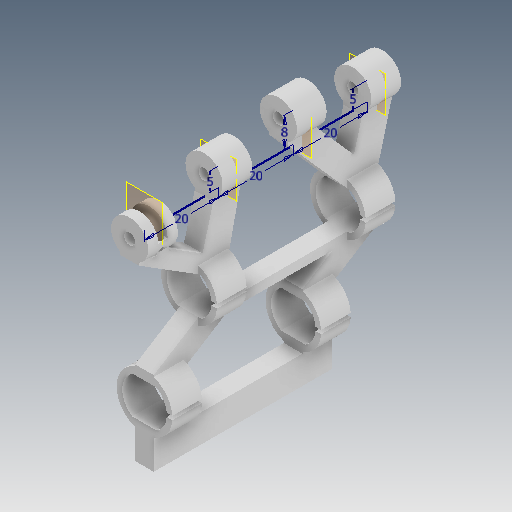
# Autodesk Inventor part: base_hand
Saved by Autodesk Inventor 2020.2 (Build 242310000, 310)
## iProperties
Created: 2020-04-08
Part Number: base_hand
Material: Generic
Document SubType Name: Modeling
Designer: Bardo91
Density: 1 g/cm^3
Appearance: Default
Author: Bardo91
Autodesk Inventor part; units mm, degrees
ref_plane "YZ Plane" through (0, 0, 0) normal (1, 0, 0) x (0, 1, 0)
ref_plane "XZ Plane" through (0, 0, 0) normal (0, 1, 0) x (-1, 0, 0)
sketch "Sketch1" plane through (0, 0, 0) normal (1, 0, 0) x (0, 1, 0)
  line L0 (0, 0) -> (0, -20)
  line L1 (0, -20) -> (0, -40)
  line L2 (0, -40) -> (0, -60)
  line L3 (0, -20) -> (5, -20)
  line L4 (0, -40) -> (8, -40)
  line L5 (0, -60) -> (5, -60)
  dimension "d0" = 20
  dimension "d1" = 20
  dimension "d2" = 20
  dimension "d4" = 5
  dimension "d5" = 8
  dimension "d6" = 5
  constraints: 12 end point, 2 horizontal, 2 point on line, 1 perpendicular, 1 vertical
  measures "d0" distance of L0.start L0.end
  measures "d1" distance of L0.end L1.end
  measures "d2" distance of L1.end L2.end
  measures "d4" distance of L0.end L3.end
  measures "d5" distance of L1.end L4.end
  measures "d6" distance of L2.end L5.end
ref_plane "Work Plane1" through (0, 5, -20) normal (0, 0, 1) x (1, 0, 0)
ref_plane "Work Plane3" through (0, 5, -60) normal (0, 0, 1) x (1, 0, 0)
ref_plane "Work Plane2" through (0, 8, -40) normal (0, 0, 1) x (1, 0, 0)
ref_plane "Work Plane4" through (0, 0, 0) normal (0, 0, 1) x (1, 0, 0)
sketch "Sketch2" plane through (0, 0, 0) normal (0, 0, 1) x (1, 0, 0)
  circle A0 centre (0, 0) radius 1.5
  circle A1 centre (0, 0) radius 5
  dimension "d7" = 3
  dimension "d8" = 10
  constraints: 2 centre point, 2 coincident
  measures "d7" diameter of A0
  measures "d8" diameter of A1
sketch "Sketch3" plane through (0, 5, -20) normal (0, 0, 1) x (1, 0, 0)
  circle A0 centre (0, 0) radius 1.5
  circle A1 centre (0, 0) radius 5
  point P0 (0, -5)
  dimension "d9" = 3
  dimension "d10" = 10
  constraints: 2 centre point, 1 coincident
  measures "d9" diameter of A0
  measures "d10" diameter of A1
sketch "Sketch4" plane through (0, 8, -40) normal (0, 0, 1) x (1, 0, 0)
  circle A0 centre (0, 0) radius 1.5
  circle A1 centre (0, 0) radius 5
  point P0 (0, -8)
  dimension "d11" = 3
  dimension "d12" = 10
  constraints: 2 centre point, 1 coincident
  measures "d11" diameter of A0
  measures "d12" diameter of A1
sketch "Sketch5" plane through (0, 5, -60) normal (0, 0, 1) x (1, 0, 0)
  circle A0 centre (0, 0) radius 1.5
  circle A1 centre (0, 0) radius 5
  point P0 (0, -5)
  dimension "d13" = 3
  dimension "d14" = 10
  constraints: 2 centre point, 1 coincident
  measures "d13" diameter of A0
  measures "d14" diameter of A1
extrude "pinky_joint" add sketch "Sketch2" along normal mid plane 8
extrude "ring_joint" add sketch "Sketch3" along normal mid plane 8
extrude "middle_joint" add sketch "Sketch4" along normal mid plane 8
extrude "index_joint" add sketch "Sketch5" along normal mid plane 8
sketch "Sketch6" plane through (0, 0, 0) normal (0, 0, 1) x (1, 0, 0)
  circle A0 centre (0, 0) radius 1.5 projected
  line L0 (0, 0) -> (0, -20)
  line L1 (0, -20) -> (0, -40)
  circle A1 centre (0, -40) radius 6
  circle A2 centre (0, -40) radius 7.5
  line L2 (0, -40) -> (0, -35)
  line L3 (0, -35) -> (3.3166, -35)
  line L4 (0, -35) -> (-3.3166, -35)
  line L5 (0, -40) -> (0, -45)
  line L6 (0, -45) -> (3.3166, -45)
  line L7 (0, -45) -> (-3.3166, -45)
  line L8 (0, -40) -> (0, -40.5)
  line L9 (0, -40) -> (0, -39.5)
  line L10 (0, -39.5) -> (7.4833, -39.5)
  line L11 (0, -40.5) -> (7.4833, -40.5)
  point P0 (5.9791, -39.5)
  point P1 (5.9791, -40.5)
  dimension "d23" = 20
  dimension "d24" = 20
  dimension "d25" = 12
  dimension "d26" = 15
  dimension "d27" = 5
  dimension "d28" = 5
  dimension "d29" = 0.5
  dimension "d30" = 0.5
  constraints: 24 end point, 7 point on line, 6 point on circle, 3 perpendicular, 2 centre point, 2 coincident, 1 parallel, 1 vertical
  measures "d23" distance of L0.start L0.end
  measures "d24" distance of L0.end L1.end
  measures "d25" diameter of A1
  measures "d26" diameter of A2
  measures "d27" distance of L2.start L2.end
  measures "d28" distance of L2.start L5.end
  measures "d29" distance of L2.start L8.end
  measures "d30" distance of L2.start L9.end
extrude "ring_motor" add sketch "Sketch6" against normal blind 8 contours L4 A1 L1 | L1 A1 L3 | A1 L11 A2 L1 | L1 A2 L10 A1 | L7 L6 A1
sketch "Sketch7" plane through (0, 5, -20) normal (0, 0, 1) x (1, 0, 0)
  circle A0 centre (0, -5) radius 5 projected
  line L0 (0, -5) -> (0, -25)
  circle A1 centre (0, -25) radius 6
  circle A2 centre (0, -25) radius 7.5
  line L1 (0, -25) -> (0, -24.5)
  line L2 (0, -25) -> (0, -25.5)
  line L3 (0, -25.5) -> (7.4833, -25.5)
  line L4 (0, -24.5) -> (7.4833, -24.5)
  line L5 (0, -25) -> (0, -20)
  line L6 (0, -20) -> (3.3166, -20)
  line L7 (0, -20) -> (-3.3166, -20)
  line L8 (0, -25) -> (0, -30)
  line L9 (0, -30) -> (3.3166, -30)
  line L10 (0, -30) -> (-3.3166, -30)
  point P0 (5.9791, -24.5)
  point P1 (5.9791, -25.5)
  dimension "d33" = 20
  dimension "d34" = 12
  dimension "d35" = 15
  dimension "d36" = 0.5
  dimension "d37" = 0.5
  dimension "d50" = 5
  dimension "d51" = 5
  constraints: 22 end point, 6 point on circle, 5 point on line, 3 perpendicular, 2 centre point, 2 coincident, 2 vertical
  measures "d33" distance of L0.start L0.end
  measures "d34" diameter of A1
  measures "d35" diameter of A2
  measures "d36" distance of L1.start L1.end
  measures "d37" distance of L1.start L2.end
  measures "d50" distance of L1.start L5.end
  measures "d51" distance of L1.start L8.end
extrude "pinky_motor" add sketch "Sketch7" along normal blind 8 contours L7 A1 L0 | L0 A1 L6 | A1 L3 A2 L0 | L0 A2 L4 A1 | L10 L9 A1
sketch "Sketch8" plane through (0, 8, -40) normal (0, 0, 1) x (1, 0, 0)
  circle A0 centre (0, -8) radius 1.5 projected
  arc A1 (5.9791, -27.5) -> (5.9791, -28.5) centre (0, -28) ccw projected
  line L0 (0, -8) -> (0, -28)
  line L1 (0, -28) -> (0, -48)
  circle A2 centre (0, -48) radius 6
  circle A3 centre (0, -48) radius 7.5
  line L2 (0, -48) -> (0, -48.5)
  line L3 (5.9791, -48.5) -> (7.4833, -48.5) projected
  line L4 (0, -48.5) -> (7.4833, -48.5)
  line L5 (0, -48) -> (0, -47.5)
  arc A4 (7.4833, -47.5) -> (7.4833, -48.5) centre (0, -48) ccw projected
  line L6 (0, -47.5) -> (7.4833, -47.5)
  line L7 (0, -48) -> (0, -53)
  line L8 (0, -53) -> (3.3166, -53)
  arc A5 (5.9791, -47.5) -> (5.9791, -48.5) centre (0, -48) ccw projected
  line L9 (0, -53) -> (-3.3166, -53)
  line L10 (0, -48) -> (0, -43)
  line L11 (0, -43) -> (-3.3166, -43)
  line L12 (0, -43) -> (3.3166, -43)
  point P0 (3.3166, -53)
  point P1 (-3.3166, -53)
  point P2 (-3.3166, -43)
  point P3 (3.3166, -43)
  point P4 (0.7483, -48)
  point P5 (0, -48)
  point P6 (0, -48)
  point P7 (-5.4544, -45.5)
  point P8 (6.4575, -44.1854)
  point P9 (6, -43.5)
  point P10 (5.9867, -43.5)
  point P11 (5.4544, -45.5)
  point P12 (-5.9812, -43.475)
  point P13 (5.9955, -43.4941)
  dimension "d40" = 20
  dimension "d41" = 20
  dimension "d42" = 12
  dimension "d43" = 15
  dimension "d44" = 0.5
  dimension "d45" = 0.5
  dimension "d46" = 5
  dimension "d47" = 5
  constraints: 24 end point, 5 point on line, 4 point on circle, 2 centre point, 2 coincident, 2 perpendicular, 2 vertical, 1 horizontal
  measures "d40" distance of L0.start L0.end
  measures "d41" distance of L0.end L1.end
  measures "d42" diameter of A2
  measures "d43" diameter of A3
  measures "d44" distance of L2.start L2.end
  measures "d45" distance of L2.start L5.end
  measures "d46" distance of L7.start L7.end
  measures "d47" distance of L10.start L10.end
extrude "index_motor" add sketch "Sketch8" against normal blind 8 contours L11 A2 L1 | L1 A2 L12 | A2 L3 A3 L1 | L1 A3 L6 A2 | L9 L8 A2
sketch "Sketch9" plane through (0, 5, -60) normal (0, 0, 1) x (1, 0, 0)
  line L0 (0, -5) -> (0, -25)
  circle A0 centre (0, -25) radius 6
  circle A1 centre (0, -25) radius 7.5
  line L1 (0, -25) -> (0, -30)
  line L2 (3.3166, -30) -> (-3.3166, -30) projected
  line L3 (0, -30) -> (3.3166, -30)
  line L4 (3.3166, -30) -> (0, -30)
  line L5 (-3.3166, -30) -> (0, -30)
  line L6 (0, -25) -> (0, -20)
  line L7 (-3.3166, -20) -> (3.3166, -20) projected
  line L8 (0, -20) -> (3.3166, -20)
  line L9 (0, -20) -> (-3.3166, -20)
  line L10 (0, -25) -> (0, -25.5)
  line L11 (7.4833, -25.5) -> (5.9791, -25.5) projected
  line L12 (0, -25.5) -> (7.4833, -25.5)
  line L13 (0, -25) -> (0, -24.5)
  arc A2 (7.4833, -24.5) -> (7.4833, -25.5) centre (0, -25) ccw projected
  line L14 (0, -24.5) -> (7.4833, -24.5)
  point P0 (5.9791, -24.5)
  dimension "d52" = 20
  dimension "d53" = 12
  dimension "d54" = 15
  dimension "d55" = 5
  dimension "d56" = 5
  dimension "d57" = 0.5
  dimension "d58" = 0.5
  constraints: 24 end point, 3 point on line, 2 centre point, 2 coincident, 2 collinear, 2 vertical, 1 midpoint, 1 perpendicular, 1 point on circle
  measures "d52" distance of L0.start L0.end
  measures "d53" diameter of A0
  measures "d54" diameter of A1
  measures "d55" distance of L1.start L1.end
  measures "d56" distance of L1.start L6.end
  measures "d57" distance of L1.start L10.end
  measures "d58" distance of L1.start L13.end
extrude "middle_motor" add sketch "Sketch9" along normal blind 8 contours L7 A0 L0 | L0 A0 L7 | A0 L11 A1 L0 | L0 A1 L14 A0 | L2 A0
sketch "Sketch16" plane through (0, 0, 0) normal (1, 0, 0) x (0, 1, 0)
  line L0 (-15, -20) -> (-15, -12) projected
  line L1 (-19.5, -12) -> (-15, -12) projected
  line L2 (-19.5, -20) -> (-15, -20) projected
  line L3 (-15, -20) -> (3.5, -24)
  line L4 (0, -24) -> (10, -24) projected
  line L5 (-15, -60) -> (-15, -52) projected
  line L6 (6.5, -36) -> (9.5, -36) projected
  line L7 (0, -64) -> (10, -64) projected
  line L8 (-5, -4) -> (5, -4) projected
  line L9 (-15, -20) -> (-5, -4)
  line L10 (10, -16) -> (0, -16) projected
  line L11 (-15, -12) -> (0, -16)
  line L12 (10, -56) -> (0, -56) projected
  line L13 (-15, -52) -> (0, -56)
  line L14 (3, -44) -> (13, -44) projected
  line L15 (3, -44) -> (-15, -60)
  line L16 (-5, -4) -> (-1.5, -4)
  line L17 (-1.5, 4) -> (-1.5, -4)
  line L18 (5, 4) -> (-5, 4) projected
  line L19 (0, -16) -> (3.5, -16)
  line L20 (6.5, -24) -> (3.5, -24) projected
  line L21 (3.5, -16) -> (3.5, -24)
  line L22 (3, -44) -> (6.5, -44)
  line L23 (-15, -12) -> (-5, 4)
  line L24 (-1.5, 4) -> (-5, 4)
  line L25 (9.5, -44) -> (6.5, -44) projected
  line L26 (3, -44) -> (6.5, -44)
  line L27 (6.5, -44) -> (6.5, -36)
  line L28 (13, -36) -> (3, -36) projected
  line L29 (3, -36) -> (6.5, -36)
  line L30 (3, -36) -> (-15, -52)
  line L31 (0, -56) -> (3.5, -56)
  line L32 (3.5, -64) -> (3.5, -56)
  line L33 (3.5, -56) -> (3.5, -64) projected
  line L34 (0, -64) -> (-15, -60)
  line L35 (-45, 0) -> (-45, -8) projected
  line L36 (-45, 0) -> (-55, 0)
  line L37 (-55, 0) -> (-55, -48)
  line L38 (-47.5, -48) -> (-32.5, -48) projected
  line L39 (-55, -48) -> (-45, -48)
  line L40 (-32.5, -40) -> (-47.5, -40) projected
  line L41 (-47.5, -8) -> (-32.5, -8) projected
  line L42 (-47.5, -40) -> (-47.5, -8)
  line L43 (-47.5, -8) -> (-45, -8)
  line L44 (-45, 0) -> (-40.5, 0) projected
  line L45 (-45, 0) -> (-45, -8)
  line L46 (-45, -40) -> (-45, -48) projected
  line L47 (-47.5, -40) -> (-45, -40)
  line L48 (-45, -40) -> (-45, -48)
  line L49 (-32.5, 0) -> (-47.5, 0) projected
  line L50 (-25, -20) -> (-25, -12) projected
  line L51 (-32.5, 0) -> (-25, -12)
  line L52 (-12.5, -20) -> (-27.5, -20) projected
  line L53 (-27.5, -20) -> (-35, -8)
  line L54 (-35, 0) -> (-35, -8) projected
  line L55 (-35, -8) -> (-35, 0)
  line L56 (-35, 0) -> (-32.5, 0)
  line L57 (-25, -12) -> (-20.5, -12) projected
  line L58 (-25, -12) -> (-25, -20)
  line L59 (-27.5, -20) -> (-25, -20)
  line L60 (-25, -60) -> (-25, -52) projected
  line L61 (-32.5, -40) -> (-25, -52)
  line L62 (-25, -52) -> (-25, -60)
  line L63 (-12.5, -60) -> (-27.5, -60) projected
  line L64 (-25, -60) -> (-27.5, -60)
  line L65 (-35, -40) -> (-35, -48) projected
  line L66 (-27.5, -60) -> (-35, -48)
  line L67 (-35, -48) -> (-35, -40)
  line L68 (-35, -40) -> (-32.5, -40)
  line L69 (-25, -20) -> (-20.5, -20) projected
  line L70 (-25, -20) -> (-25, -52)
  line L71 (-27.5, -20) -> (-27.5, -52)
  line L72 (-27.5, -60) -> (-27.5, -52) projected
  point P0 (0, 0)
  point P1 (-8.0769, -53.8462)
  point P2 (-10.7143, -13.1429)
  point P3 (-40.5, -48)
  point P4 (-39.5, -48)
  point P5 (-39.5, -40)
  point P6 (-40.5, -40)
  point P7 (-40.5, -8)
  point P8 (-39.5, -8)
  point P9 (-39.5, 0)
  point P10 (-19.5, -60)
  point P11 (-20.5, -60)
  point P12 (-27.5, -48)
  dimension "d72" = 10
  constraints: 82 end point, 9 collinear, 8 perpendicular, 8 point on line, 4 horizontal, 2 vertical, 1 parallel
  measures "d72" distance of L35.start L36.end
extrude "structure_hand" add sketch "Sketch16" along normal mid plane 5 contours L9 L11 L10 L21 L3 | L0 L11 L9 | L23 L18 L17 L8 L9 L11 | L5 L13 L15 | L15 L13 L12 L32 L7 L34 | L30 L28 L27 L14 L15 L13 | L35 L41 L42 L40 L46 L38 L39 L37 L36 | L54 L49 L51 L50 L52 L53 | L52 L70 L61 L71 | L71 L72 L66 L65 L40 L61 | L61 L60 L63 L72 L71
sketch "Sketch17" plane through (0, 0, 0) normal (0, 1, 0) x (-1, 0, 0)
  line L0 (0, 0) -> (-3.5, 0)
  line L1 (2.5, 0) -> (-2.5, 0) projected
  line L2 (0, 0) -> (3.5, 0)
  line L3 (7.5, 0) -> (2.5, 0) projected
  circle A0 centre (3.5, 0) radius 1.25
  circle A1 centre (-3.5, 0) radius 1.25
  line L4 (0, 0) -> (0, -1.1165)
  line L5 (-3.5, -1.25) -> (-5, -1.25)
  line L6 (-5, -4) -> (-5, 4) projected
  line L7 (-3.5, 1.25) -> (-5, 1.25)
  line L8 (-5, -4) -> (-5, 4) projected
  dimension "d73" = 3.5
  dimension "d74" = 3.5
  dimension "d75" = 2.5
  dimension "d76" = 2.5
  constraints: 10 end point, 3 point on line, 2 centre point, 2 coincident, 2 point on circle, 1 collinear, 1 horizontal, 1 parallel, 1 vertical
  measures "d73" distance of L0.start L0.end
  measures "d74" distance of L0.start L2.end
  measures "d75" diameter of A0
  measures "d76" diameter of A1
revolve "Revolution1" cut sketch "Sketch17" angle 180 about axis through (0, 0, 0) along (0, 0, 1) contours A1 | A1 L5 L6 L7
extrude "Extrusion10" cut sketch "Sketch17" against normal mid plane 10 contours L2 L3 A0 L1 | L1 A0 L3 L2 | A1
body "Solid1"
